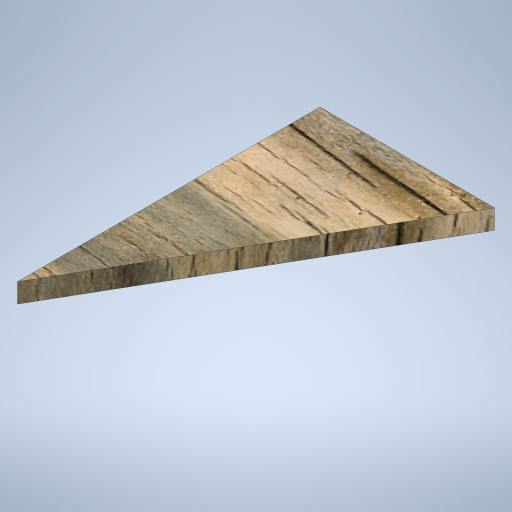
# Autodesk Inventor part: Triangle_Ocampo
Saved by Autodesk Inventor 2023 (Build 270158000, 158)
## iProperties
Created: 2025-03-05
Part Number: Triangle_Ocampo
Material: Generic
Document SubType Name: Modeling
Designer: FrameUser
Density: 1 g/cm^3
Appearance: Default
Author: FrameUser
Autodesk Inventor part; units mm, degrees
ref_plane "YZ Plane" through (0, 0, 0) normal (1, 0, 0) x (0, 1, 0)
ref_plane "XZ Plane" through (0, 0, 0) normal (0, 1, 0) x (-1, 0, 0)
ref_plane "XY Plane" through (0, 0, 0) normal (0, 0, 1) x (1, 0, 0)
sketch "Sketch1" plane through (0, 0, 0) normal (0, 1, 0) x (-1, 0, 0)
  line L0 (0, 0) -> (0, -98.9838)
  line L1 (0, -98.9838) -> (-57.15, -98.9838)
  line L2 (-57.15, -98.9838) -> (0, 0)
  dimension "d0" = 98.9838
  dimension "d1" = 57.15
  constraints: 6 end point, 1 perpendicular, 1 vertical
  measures "d0" distance of L0.start L0.end
  measures "d1" distance of L0.end L1.end
extrude "Extrusion1" add sketch "Sketch1" along normal blind 6.35
body "Solid1"
